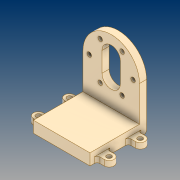
# Autodesk Inventor part: 08_Ga_dong_co
Saved by Autodesk Inventor 2021 (Build 250183000, 183)
## iProperties
Created: 2024-04-01
Part Number: 08_Ga_dong_co
Material: Polyethylene, High Density
Document SubType Name: Modeling
Designer: Admin
Density: 0.952 g/cm^3
Appearance: Smooth - Off-White
Author: Admin
Autodesk Inventor part; units mm, degrees
ref_plane "YZ Plane" through (0, 0, 0) normal (1, 0, 0) x (0, 1, 0)
ref_plane "XZ Plane" through (0, 0, 0) normal (0, 1, 0) x (-1, 0, 0)
sketch "Sketch1" plane through (0, 0, 0) normal (0, 0, 1) x (1, 0, 0)
  circle A0 centre (0, 0) radius 20
  circle A1 centre (0, 15.55) radius 1.6
  line L0 (-20, 0) -> (20, 0) construction
  line L1 (20, 0) -> (20, -33)
  line L2 (20, -33) -> (-20, -33)
  line L3 (-20, -33) -> (-20, 0)
  circle A2 centre (-13.4667, 7.775) radius 1.6
  circle A3 centre (-13.4667, -7.775) radius 1.6
  circle A4 centre (0, -15.55) radius 1.6
  circle A5 centre (13.4667, -7.775) radius 1.6
  circle A6 centre (13.4667, 7.775) radius 1.6
  line L4 (0, -7) -> (0, 7) construction
  line L5 (-6.5, -7) -> (-6.5, 7)
  line L6 (6.5, 7) -> (6.5, -7)
  arc A7 (-6.5, -7) -> (6.5, -7) centre (0, -7) ccw
  arc A8 (6.5, 7) -> (-6.5, 7) centre (0, 7) ccw
  dimension "d0" = 40
  dimension "d1" = 15.55
  dimension "d3" = 33
  dimension "d6" = 360
  dimension "d8" = 6.5
  dimension "d9" = 14
  constraints: 16 end point, 9 centre point, 6 point on circle, 5 tangent, 3 parallel, 1 coincident, 1 horizontal, 1 midpoint, 1 perpendicular, 1 vertical, 13 other
  measures "d0" diameter of A0
  measures "d1" distance of point (0, 0) A1.centre
  measures "d3" distance between parallel lines of L0 L2
  measures "d8" radius of A8
  measures "d9" distance of L6.start L6.end
extrude "Extrusion1" add sketch "Sketch1" along normal blind 5 contours A0 | L1 L2 L3 A0 | A1 | A2 | A3 | A4 | A5 | A6
sketch "Sketch2" plane through (0, 0, 0) normal (0, 0, -1) x (-1, 0, 0)
  line L0 (20, 0) -> (20, -33) projected
  arc A0 (20, 0) -> (-20, 0) centre (0, 0) ccw projected
  line L1 (-20, -33) -> (-20, 0) projected
  line L2 (20, -33) -> (-20, -33) projected
  line L3 (-6.5, 7) -> (-6.5, -7) projected
  arc A1 (6.5, 7) -> (-6.5, 7) centre (0, 7) ccw projected
  line L4 (6.5, -7) -> (6.5, 7) projected
  arc A2 (-6.5, -7) -> (6.5, -7) centre (0, -7) ccw projected
  circle A3 centre (0, 0) radius 15.5 construction
  circle A4 centre (-7.75, 13.4234) radius 1.6
  line L5 (0, 0) -> (-7.75, 13.4234) construction
  line L6 (0, 0) -> (0, 15.5) construction
  circle A5 centre (-15.5, 0) radius 1.6
  circle A6 centre (-7.75, -13.4234) radius 1.6
  circle A7 centre (7.75, -13.4234) radius 1.6
  circle A8 centre (15.5, 0) radius 1.6
  circle A9 centre (7.75, 13.4234) radius 1.6
  dimension "d12" = 31
  dimension "d13" = 3.2
  dimension "d14" = 30
  dimension "d17" = 360
  constraints: 7 centre point, 4 end point, 2 point on circle, 1 coincident, 1 vertical, 13 other
  measures "d12" diameter of A3
  measures "d13" diameter of A4
  measures "d14" angle of L6 L5
extrude "Extrusion2" cut sketch "Sketch2" against normal blind 5 contours A4 | A5 | A6 | A7 | A8 | A9
sketch "Sketch3" plane through (-20, -33, 0) normal (0, -1, 0) x (1, 0, 0)
  line L0 (0, 0) -> (40, 0) projected
  line L1 (40, 0) -> (40, 5) projected
  line L2 (0, 5) -> (40, 5) projected
  line L3 (0, 0) -> (0, 5) projected
  line L4 (40, 0) -> (40, 5) projected
  line L5 (40, 5) -> (0, 5)
  line L6 (0, 5) -> (0, 40)
  line L7 (0, 40) -> (40, 40)
  line L8 (40, 40) -> (40, 5)
  point P0 (20, 0)
  dimension "d21" = 40
  constraints: 8 end point, 3 equal length, 1 perpendicular
  measures "d21" distance between parallel lines of L0 L7
extrude "Extrusion3" add sketch "Sketch3" against normal blind 8 contours L6 L7 L8 L2
fillet "Fillet1" radius 2 1 edges at (0, -33, 0)
sketch "Sketch4" plane through (-20, -33, 2) normal (0, -1, 0) x (1, 0, 0)
  line L0 (40, 38) -> (0, 38) projected
  line L1 (0, 0) -> (0, 38) projected
  line L2 (40, 0) -> (0, 0) projected
  line L3 (40, 0) -> (40, 38) projected
  line L4 (5, 4) -> (-5, 4)
  line L5 (-5, 4) -> (-5, 11)
  line L6 (-5, 11) -> (5, 11)
  line L7 (5, 11) -> (5, 4)
  line L8 (5, 4) -> (-5, 11) construction
  line L9 (-5, 4) -> (5, 11) construction
  circle A0 centre (-5, 7.5) radius 3.5
  circle A1 centre (-5, 7.5) radius 1.75
  point P0 (20, -2)
  point P1 (0, 7.5)
  point P2 (0, 4)
  point P3 (0, 11)
  point P4 (-5, 11)
  dimension "d26" = 7
  dimension "d27" = 5
  dimension "d28" = 4
  dimension "d29" = 3.5
  constraints: 12 end point, 3 midpoint, 2 parallel, 2 perpendicular, 1 centre point, 1 coincident, 1 point on line, 3 other
  measures "d27" distance between parallel lines of L1 L5
  measures "d28" distance between parallel lines of L2 L4
  measures "d29" diameter of A1
extrude "Extrusion4" add sketch "Sketch4" against normal blind 4 contours L1 L4 A0 L6 | A0 L5 A1 | L5 A1 A0
ref_plane "Work Plane1" through (0, 0, 22.5) normal (0, 0, 1) x (1, 0, 0)
ref_plane "Work Plane2" through (0, 0, 20.5) normal (0, 0, 1) x (1, 0, 0)
mirror "Mirror2" about plane through (0, 0, 0) normal (1, 0, 0) of "Extrusion4"
mirror "Mirror3" about plane through (0, 0, 20.5) normal (0, 0, 1) of "Extrusion4", "Mirror2"
fillet "Fillet4" radius 2 8 edges at (20, -31, 6) (20, -31, 28) (-20, -31, 6) (-20, -31, 13) (-20, -31, 28) (-20, -31, 35) (20, -31, 35) (20, -31, 13)
body "Solid1"
